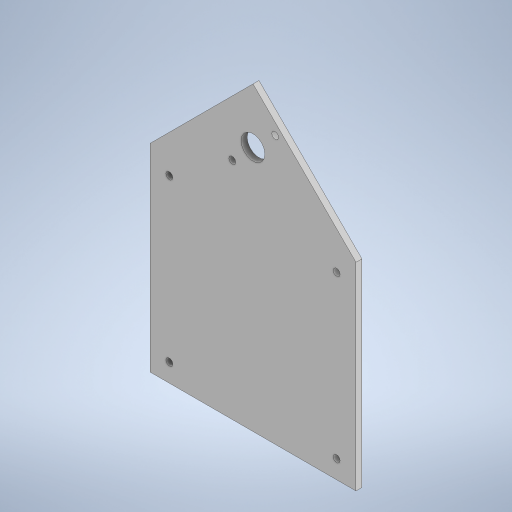
# Autodesk Inventor part: DekselCase
Saved by Autodesk Inventor 2023 (Build 270158000, 158)
## iProperties
Created: 2023-05-29
Part Number: DekselCase
Material: Generic
Document SubType Name: Modeling
Designer: jaspe
Density: 1 g/cm^3
Appearance: Default
Author: jaspe
Autodesk Inventor part; units mm, degrees
ref_plane "YZ Plane" through (0, 0, 0) normal (1, 0, 0) x (0, 1, 0)
ref_plane "XZ Plane" through (0, 0, 0) normal (0, 1, 0) x (-1, 0, 0)
ref_plane "XY Plane" through (0, 0, 0) normal (0, 0, 1) x (1, 0, 0)
sketch "Sketch2" plane through (0, 0, 0) normal (0, 0, 1) x (1, 0, 0)
  line L0 (0, 0) -> (104, 0)
  line L1 (104, 0) -> (104, 100)
  line L2 (104, 100) -> (0, 100)
  line L3 (0, 100) -> (0, 0)
  line L4 (0, 100) -> (52, 152)
  line L5 (0, 100) -> (73.5391, 100) construction
  line L6 (52, 152) -> (104, 100)
  line L7 (9.75, 100) -> (9.75, 0)
  line L8 (94.25, 100) -> (94.25, 0)
  circle A0 centre (9.75, 9.25) radius 1.75
  circle A1 centre (9.75, 90.75) radius 1.75
  line L9 (9.75, 90.75) -> (94.25, 90.75)
  line L10 (9.75, 9.25) -> (94.25, 9.25)
  circle A2 centre (94.25, 90.75) radius 1.75
  circle A3 centre (94.25, 9.25) radius 1.75
  dimension "d0" = 104
  dimension "d1" = 100
  dimension "d2" = 45
  dimension "d3" = 73.5391
  dimension "d4" = 9.75
  dimension "d5" = 9.75
  dimension "d6" = 9.25
  dimension "d7" = 90.75
  dimension "d8" = 3.5
  dimension "d9" = 3.5
  dimension "d10" = 3.5
  dimension "d11" = 3.5
  constraints: 22 end point, 8 point on line, 5 perpendicular, 4 centre point, 3 horizontal, 2 coincident, 2 parallel, 1 equal length
  measures "d0" distance of L2.end L1.end
  measures "d1" distance of L2.end L0.start
  measures "d2" angle of L5 L4
  measures "d3" distance of L2.end L4.end
  measures "d4" distance between parallel lines of L7 L3
  measures "d5" distance between parallel lines of L8 L1
  measures "d6" distance from line of L0 L10.start
  measures "d7" distance from line of L0 L9.start
  measures "d8" diameter of A1
  measures "d9" diameter of A0
  measures "d10" diameter of A3
  measures "d11" diameter of A2
extrude "Extrusion1" add sketch "Sketch2" against normal blind 3 contours L3 L2 L7 A1 A0 L0 | L7 A0 L10 A3 L8 L0 | L4 L6 L2 | L8 A3 A2 L2 L1 L0 | L2 L8 A2 L9 A1 L7 | L7 A1 L9 A2 L8 A3 L10 A0
sketch "Sketch3" plane through (0, 0, 0) normal (0, 0, 1) x (1, 0, 0)
  line L0 (0, 100) -> (52, 152) projected
  line L1 (52, 152) -> (52, 0)
  circle A0 centre (52, 124.2497) radius 6
  line L2 (41.5364, 135.0719) -> (63.181, 135.0719)
  line L3 (63.181, 135.0719) -> (63.181, 113.4274)
  line L4 (63.181, 113.4274) -> (41.5364, 113.4274)
  line L5 (41.5364, 113.4274) -> (41.5364, 135.0719)
  circle A1 centre (63.181, 135.0719) radius 1.727
  circle A2 centre (41.5364, 113.4274) radius 1.727
  point P0 (0, 0)
  point P1 (52.3587, 113.4274)
  dimension "d14" = 12
  dimension "d18" = 30.61
  dimension "d19" = 3.454
  dimension "d20" = 3.454
  dimension "d21" = 10.8223
  constraints: 10 end point, 3 centre point, 2 coincident, 2 parallel, 2 perpendicular, 1 horizontal, 1 midpoint, 1 point on line, 1 vertical
  measures "d14" diameter of A0
  measures "d18" distance of L2.end L4.end
  measures "d19" diameter of A1
  measures "d20" diameter of A2
  measures "d21" vertical distance of point (52.359, 113.427) A0.centre
extrude "Extrusion2" cut sketch "Sketch3" against normal blind 3 contours A0 L1 | L1 A0 | A1 L3 L2 | L2 L3 A1 | A2 L4 L5 | L5 L4 A2
body "Solid1"
